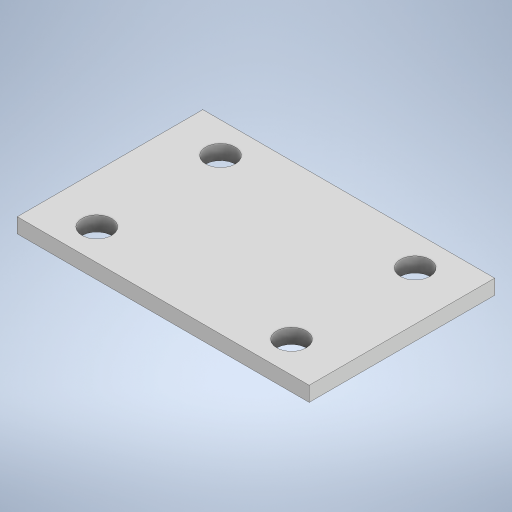
# Autodesk Inventor part: SensorBoxBraket
Saved by Autodesk Inventor 2024.2 (Build 282272000, 272)
## iProperties
Created: 2024-02-07
Part Number: SensorBoxBraket
Material: Generic
Document SubType Name: Sheet Metal
Designer: airso
Density: 1 g/cm^3
Sheet Metal Rule: Default
Appearance: Default
Author: airso
Autodesk Inventor part; units mm, degrees
ref_plane "YZ Plane" through (0, 0, 0) normal (1, 0, 0) x (0, 1, 0)
ref_plane "XZ Plane" through (0, 0, 0) normal (0, 1, 0) x (-1, 0, 0)
ref_plane "XY Plane" through (0, 0, 0) normal (0, 0, 1) x (1, 0, 0)
sketch "Sketch1" plane through (0, 0, 0) normal (0, 1, 0) x (-1, 0, 0)
  line L0 (0, 0) -> (-59.944, 0)
  line L1 (-59.944, 0) -> (-59.944, -38.1)
  line L2 (-59.944, -38.1) -> (0, -38.1)
  line L3 (0, -38.1) -> (0, 0)
  dimension "d0" = 59.944
  dimension "d1" = 38.1
  measures "d0" distance of L2.end L1.end
  measures "d1" distance of L2.end L0.start
extrude "Plate1" add sketch "Sketch1" along normal blind 3.048
sketch "Sketch3" plane through (0, 3.048, 0) normal (0, 1, 0) x (1, 0, 0)
  line L0 (0, 0) -> (59.944, 0) projected
  line L1 (50.8, 0) -> (50.8, 38.1)
  line L2 (0, 0) -> (0, 38.1) projected
  line L3 (0, 38.1) -> (59.944, 38.1) projected
  line L4 (59.944, 38.1) -> (59.944, 0) projected
  point P0 (9.9822, 6.35)
  point P1 (9.9822, 31.75)
  point P2 (49.9618, 31.75)
  point P3 (49.9618, 6.35)
  dimension "d4" = 38.1
  dimension "d5" = 50.8
  dimension "d6" = 6.35
  dimension "d7" = 9.9822
  dimension "d8" = 9.9822
  dimension "d9" = 6.35
  dimension "d10" = 6.35
  dimension "d11" = 6.35
  dimension "d12" = 9.9822
  dimension "d13" = 9.9822
  constraints: 2 end point, 1 point on line, 1 vertical
  measures "d4" distance of L1.start L1.end
  measures "d5" distance between parallel lines of L2 L1
  measures "d6" distance from line of L3 point (9.982, 31.75)
  measures "d7" distance from line of point (9.982, 31.75) L2
  measures "d8" distance from line of L2 point (9.982, 6.35)
  measures "d9" distance from line of L0 point (9.982, 6.35)
  measures "d10" distance from line of L3 point (49.962, 31.75)
  measures "d11" distance from line of L0 point (49.962, 6.35)
  measures "d12" distance from line of L4 point (49.962, 6.35)
  measures "d13" distance from line of L4 point (49.962, 31.75)
hole "Hole1" at (9.9822, 3.048, -6.35) at (9.9822, 3.048, -31.75) at (49.9618, 3.048, -31.75) at (49.9618, 3.048, -6.35) direction (0, -1, 0) diameter 6.096 end through all
equation "\"d19\" = Thickness"
equation "\"d2\" = Thickness"
equation "\"BendRadius\" = Thickness"
equation "\"BendReliefWidth\" = Thickness"
equation "\"BendReliefDepth\" = 0.5 * Thickness"
equation "\"CornerReliefSize\" = 4 * Thickness"
equation "\"MinimumRemnant\" = 2 * Thickness"
equation "\"TransitionRadius\" = BendRadius"
equation "\"JacobiRadiusSize\" = BendRadius"
equation "\"GapSize\" = Thickness"
equation "\"Thickness\" = 3.048"
body "Solid1"
